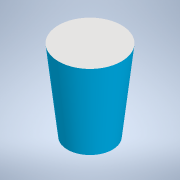
# Autodesk Inventor part: 杯子
Saved by Autodesk Inventor 2020 (Build 240168000, 168)
## iProperties
Created: 2023-03-07
Part Number: 杯子
Material: 一般
Document SubType Name: Modeling
Designer: robot
Density: 1 g/cm^3
Appearance: 預設
Mass: 256.825 g
Surface Area: 228.809 cm^2
Volume: 256.825 cm^3
Author: robot
Autodesk Inventor part; units mm, degrees
ref_plane "YZ Plane" through (0, 0, 0) normal (1, 0, 0) x (0, 1, 0)
ref_plane "XZ Plane" through (0, 0, 0) normal (0, 1, 0) x (-1, 0, 0)
ref_plane "XY Plane" through (0, 0, 0) normal (0, 0, 1) x (1, 0, 0)
sketch "草圖1" plane through (0, 0, 0) normal (0, 1, 0) x (-1, 0, 0)
  point P0 (0, 0)
sketch "草圖2" plane through (0, 0, 0) normal (0, 0, 1) x (1, 0, 0)
  line L0 (0, 0) -> (25, 0)
  line L1 (25, 0) -> (18.1781, 0)
  line L2 (0, 0) -> (0, 90)
  line L3 (0, 90) -> (35, 90)
  line L4 (35, 90) -> (25, 0)
  dimension "d0" = 25
  dimension "d1" = 90
  dimension "d2" = 35
  constraints: 10 end point, 2 horizontal, 1 point on line, 1 vertical
  measures "d0" distance of L0.start L0.end
  measures "d1" distance of L0.start L2.end
  measures "d2" distance of L2.end L3.end
revolve "迴轉1" add sketch "草圖2" angle 360 about axis through (0, 0, 0) along (0, 1, 0)
